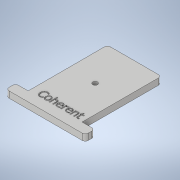
# Autodesk Inventor part: 00_Slider_Mask_DPC
Saved by Autodesk Inventor 2022 (Build 260153000, 153)
## iProperties
Created: 2021-10-22
Part Number: 00_Slider_Mask_DPC
Material: Generic
Document SubType Name: Modeling
Designer: diederichbenedict
Density: 1 g/cm^3
Appearance: Default
Author: diederichbenedict
Autodesk Inventor part; units mm, degrees
ref_plane "YZ Plane" through (0, 0, 0) normal (1, 0, 0) x (0, 1, 0)
ref_plane "XZ Plane" through (0, 0, 0) normal (0, 1, 0) x (-1, 0, 0)
ref_plane "XY Plane" through (0, 0, 0) normal (0, 0, 1) x (1, 0, 0)
sketch "Sketch1" plane through (0, 0, 0) normal (0, 1, 0) x (-1, 0, 0)
  line L0 (-17, 25) -> (17, 25)
  line L1 (17, 25) -> (17, -25)
  line L2 (17, -25) -> (-17, -25)
  line L3 (-17, -25) -> (-17, 25)
  line L4 (-17, 25) -> (17, -25) construction
  line L5 (17, 25) -> (-17, -25) construction
  line L6 (9, -17) -> (9, 17)
  line L7 (9, 17) -> (-9, 17)
  line L8 (-9, 17) -> (-9, -17)
  line L9 (-9, -17) -> (9, -17)
  line L10 (-25, 31) -> (25, 31)
  line L11 (25, 31) -> (25, 25)
  line L12 (25, 25) -> (-25, 25)
  line L13 (-25, 25) -> (-25, 31)
  line L14 (-25, 31) -> (25, 25) construction
  line L15 (25, 31) -> (-25, 25) construction
  point P0 (0, 0)
  point P1 (0, 28)
  point P2 (0, 25)
  dimension "d0" = 34
  dimension "d1" = 50
  dimension "d2" = 8
  dimension "d3" = 50
  dimension "d4" = 6
  constraints: 32 end point, 6 midpoint, 6 parallel, 3 perpendicular, 2 horizontal, 3 other
  measures "d0" distance of L1.end L2.end
  measures "d1" distance of L0.end L1.end
  measures "d2" distance between parallel lines of L1 L6
  measures "d3" distance of L11.end L12.end
  measures "d4" distance of L10.end L11.end
extrude "Extrusion1" add sketch "Sketch1" along normal blind 4 contours L12 L13 L10 L11 L0 | L0 L1 L2 L3 | L9 L8 L7 L6
sketch "Sketch2" plane through (0, 4, 0) normal (0, 1, 0) x (1, 0, 0)
  line L0 (25, -25) -> (17, -25) projected
  line L1 (17, -25) -> (17, 25) projected
  line L2 (17, 25) -> (-17, 25) projected
  line L3 (-17, 25) -> (-17, -25) projected
  line L4 (-17, -25) -> (-25, -25) projected
  line L5 (-25, -25) -> (-25, -31) projected
  line L6 (-25, -31) -> (25, -31) projected
  line L7 (25, -31) -> (25, -25) projected
  line L8 (13.5, 17) -> (-13.5, 17)
  line L9 (13.5, 17) -> (-13.5, -17) construction
  line L10 (-13.5, 17) -> (13.5, -17) construction
  circle A0 centre (0, 0.2783) radius 1.5
  point P0 (-1.4697, 0.3)
  point P1 (1.4697, 0.3)
  point P2 (-1.5, 0.2783)
  point P3 (1.5, 0.2783)
  dimension "d7" = 27
  dimension "d8" = 34
  dimension "d17" = 3
  constraints: 6 end point, 2 point on circle, 1 centre point, 1 horizontal
  measures "d7" distance of L10.end L9.end
  measures "d8" distance of L9.end L8.end
  measures "d17" diameter of A0
extrude "Extrusion2" cut sketch "Sketch2" against normal through all contours A0
sketch "Sketch3" plane through (0, 4, 0) normal (0, 1, 0) x (1, 0, 0)
  line L0 (-12.5562, -19.3436) -> (12.6697, -19.3436) construction
  line L1 (12.6697, -19.3436) -> (12.6697, -24.5308) construction
  line L2 (12.6697, -24.5308) -> (-12.5562, -24.5308) construction
  line L3 (-12.5562, -24.5308) -> (-12.5562, -19.3436) construction
  spline S0 degree 2 poles (-10.1618, -24.515) (-10.6351, -24.515) (-11.4359, -24.1955) (-11.7278, -23.876) knots 0 0 0 1 2 2 2
  spline S1 degree 2 poles (-11.7278, -23.876) (-12.0197, -23.5604) (-12.3392, -22.6137) (-12.3392, -21.9984) knots 0 0 0 1 2 2 2
  spline S2 degree 2 poles (-12.3392, -21.9984) (-12.3392, -21.387) (-12.0276, -20.4797) (-11.7317, -20.1444) knots 0 0 0 1 2 2 2
  spline S3 degree 2 poles (-11.7317, -20.1444) (-11.4398, -19.817) (-10.643, -19.4738) (-10.1499, -19.4738) knots 0 0 0 1 2 2 2
  spline S4 degree 2 poles (-10.1499, -19.4738) (-9.9054, -19.4738) (-9.4754, -19.5448) (-9.294, -19.6) knots 0 0 0 1 2 2 2
  spline S5 degree 2 poles (-9.294, -19.6) (-9.1362, -19.6513) (-8.8088, -19.7973) (-8.647, -19.8841) knots 0 0 0 1 2 2 2
  line L4 (-8.647, -19.8841) -> (-8.647, -20.6651)
  line L5 (-8.647, -20.6651) -> (-8.6983, -20.6651)
  spline S6 degree 2 poles (-8.6983, -20.6651) (-8.7851, -20.5862) (-9.0533, -20.3653) (-9.2466, -20.2588) knots 0 0 0 1 2 2 2
  spline S7 degree 2 poles (-9.2466, -20.2588) (-9.432, -20.1562) (-9.8699, -20.0261) (-10.1539, -20.0261) knots 0 0 0 1 2 2 2
  spline S8 degree 2 poles (-10.1539, -20.0261) (-10.4655, -20.0261) (-11.0217, -20.2825) (-11.2308, -20.527) knots 0 0 0 1 2 2 2
  spline S9 degree 2 poles (-11.2308, -20.527) (-11.4359, -20.7755) (-11.6647, -21.529) (-11.6647, -21.9984) knots 0 0 0 1 2 2 2
  spline S10 degree 2 poles (-11.6647, -21.9984) (-11.6647, -22.4993) (-11.4241, -23.2212) (-11.215, -23.4697) knots 0 0 0 1 2 2 2
  spline S11 degree 2 poles (-11.215, -23.4697) (-11.0099, -23.7103) (-10.4616, -23.9549) (-10.1539, -23.9549) knots 0 0 0 1 2 2 2
  spline S12 degree 2 poles (-10.1539, -23.9549) (-9.8738, -23.9549) (-9.3965, -23.8168) (-9.2111, -23.7143) knots 0 0 0 1 2 2 2
  spline S13 degree 2 poles (-9.2111, -23.7143) (-9.0336, -23.6117) (-8.7693, -23.3987) (-8.6944, -23.3238) knots 0 0 0 1 2 2 2
  line L6 (-8.6944, -23.3238) -> (-8.647, -23.3238)
  line L7 (-8.647, -23.3238) -> (-8.647, -24.0969)
  spline S14 degree 2 poles (-8.647, -24.0969) (-8.8088, -24.1719) (-9.0928, -24.3099) (-9.294, -24.373) knots 0 0 0 1 2 2 2
  spline S15 degree 2 poles (-9.294, -24.373) (-9.507, -24.444) (-9.8699, -24.515) (-10.1618, -24.515) knots 0 0 0 1 2 2 2
  spline S16 degree 2 poles (-5.089, -22.6019) (-5.089, -23.5249) (-5.9765, -24.5308) (-6.7181, -24.5308) knots 0 0 0 1 2 2 2
  spline S17 degree 2 poles (-6.7181, -24.5308) (-7.4794, -24.5308) (-8.3512, -23.4934) (-8.3512, -22.6019) knots 0 0 0 1 2 2 2
  spline S18 degree 2 poles (-8.3512, -22.6019) (-8.3512, -21.6868) (-7.4518, -20.673) (-6.7181, -20.673) knots 0 0 0 1 2 2 2
  spline S19 degree 2 poles (-6.7181, -20.673) (-5.9765, -20.673) (-5.089, -21.6828) (-5.089, -22.6019) knots 0 0 0 1 2 2 2
  spline S20 degree 2 poles (-5.7241, -22.6019) (-5.7241, -21.8919) (-6.2408, -21.2016) (-6.7181, -21.2016) knots 0 0 0 1 2 2 2
  spline S21 degree 2 poles (-6.7181, -21.2016) (-7.1954, -21.2016) (-7.7161, -21.8919) (-7.7161, -22.6019) knots 0 0 0 1 2 2 2
  spline S22 degree 2 poles (-7.7161, -22.6019) (-7.7161, -23.2922) (-7.1954, -24.0022) (-6.7181, -24.0022) knots 0 0 0 1 2 2 2
  spline S23 degree 2 poles (-6.7181, -24.0022) (-6.2448, -24.0022) (-5.7241, -23.304) (-5.7241, -22.6019) knots 0 0 0 1 2 2 2
  line L8 (-1.5901, -24.4283) -> (-2.2055, -24.4283)
  line L9 (-2.2055, -24.4283) -> (-2.2055, -22.3455)
  spline S24 degree 2 poles (-2.2055, -22.3455) (-2.2055, -22.093) (-2.2528, -21.6591) (-2.3238, -21.529) knots 0 0 0 1 2 2 2
  spline S25 degree 2 poles (-2.3238, -21.529) (-2.3988, -21.3909) (-2.667, -21.2568) (-2.8958, -21.2568) knots 0 0 0 1 2 2 2
  spline S26 degree 2 poles (-2.8958, -21.2568) (-3.1246, -21.2568) (-3.6098, -21.5014) (-3.8425, -21.6986) knots 0 0 0 1 2 2 2
  line L10 (-3.8425, -21.6986) -> (-3.8425, -24.4283)
  line L11 (-3.8425, -24.4283) -> (-4.4579, -24.4283)
  line L12 (-4.4579, -24.4283) -> (-4.4579, -19.3436)
  line L13 (-4.4579, -19.3436) -> (-3.8425, -19.3436)
  line L14 (-3.8425, -19.3436) -> (-3.8425, -21.1818)
  spline S27 degree 2 poles (-3.8425, -21.1818) (-3.5664, -20.9333) (-3.0339, -20.673) (-2.7341, -20.673) knots 0 0 0 1 2 2 2
  spline S28 degree 2 poles (-2.7341, -20.673) (-2.1976, -20.673) (-1.5901, -21.383) (-1.5901, -22.0575) knots 0 0 0 1 2 2 2
  line L15 (-1.5901, -22.0575) -> (-1.5901, -24.4283)
  spline S29 degree 2 poles (0.8595, -24.5111) (-0.0162, -24.5111) (-0.9787, -23.5289) (-0.9787, -22.6216) knots 0 0 0 1 2 2 2
  spline S30 degree 2 poles (-0.9787, -22.6216) (-0.9787, -21.7301) (-0.0438, -20.673) (0.7096, -20.673) knots 0 0 0 1 2 2 2
  spline S31 degree 2 poles (0.7096, -20.673) (1.0488, -20.673) (1.5735, -20.8702) (1.7667, -21.0793) knots 0 0 0 1 2 2 2
  spline S32 degree 2 poles (1.7667, -21.0793) (1.964, -21.2883) (2.173, -21.8919) (2.173, -22.3297) knots 0 0 0 1 2 2 2
  line L16 (2.173, -22.3297) -> (2.173, -22.665)
  line L17 (2.173, -22.665) -> (-0.3555, -22.665)
  spline S33 degree 2 poles (-0.3555, -22.665) (-0.3555, -23.3001) (0.2836, -23.9746) (0.8516, -23.9746) knots 0 0 0 1 2 2 2
  spline S34 degree 2 poles (0.8516, -23.9746) (1.0528, -23.9746) (1.4433, -23.8839) (1.6011, -23.8129) knots 0 0 0 1 2 2 2
  spline S35 degree 2 poles (1.6011, -23.8129) (1.7667, -23.734) (1.9955, -23.5959) (2.0705, -23.5328) knots 0 0 0 1 2 2 2
  line L18 (2.0705, -23.5328) -> (2.106, -23.5328)
  line L19 (2.106, -23.5328) -> (2.106, -24.2034)
  spline S36 degree 2 poles (2.106, -24.2034) (1.9995, -24.2468) (1.676, -24.373) (1.5498, -24.4085) knots 0 0 0 1 2 2 2
  spline S37 degree 2 poles (1.5498, -24.4085) (1.3723, -24.4598) (1.0804, -24.5111) (0.8595, -24.5111) knots 0 0 0 1 2 2 2
  spline S38 degree 2 poles (1.5735, -22.1956) (1.5656, -21.9471) (1.463, -21.5842) (1.3644, -21.4619) knots 0 0 0 1 2 2 2
  spline S39 degree 2 poles (1.3644, -21.4619) (1.2579, -21.3238) (0.9226, -21.1779) (0.6741, -21.1779) knots 0 0 0 1 2 2 2
  spline S40 degree 2 poles (0.6741, -21.1779) (0.4295, -21.1779) (0.0863, -21.3238) (-0.0557, -21.4659) knots 0 0 0 1 2 2 2
  spline S41 degree 2 poles (-0.0557, -21.4659) (-0.1937, -21.6118) (-0.3357, -21.9629) (-0.3555, -22.1956) knots 0 0 0 1 2 2 2
  line L20 (-0.3555, -22.1956) -> (1.5735, -22.1956)
  line L21 (4.7331, -21.4343) -> (4.7015, -21.4343)
  spline S42 degree 2 poles (4.7015, -21.4343) (4.6305, -21.4146) (4.4767, -21.4067) (4.3702, -21.4067) knots 0 0 0 1 2 2 2
  spline S43 degree 2 poles (4.3702, -21.4067) (4.1217, -21.4067) (3.6325, -21.6236) (3.4116, -21.8366) knots 0 0 0 1 2 2 2
  line L22 (3.4116, -21.8366) -> (3.4116, -24.4283)
  line L23 (3.4116, -24.4283) -> (2.7963, -24.4283)
  line L24 (2.7963, -24.4283) -> (2.7963, -20.7755)
  line L25 (2.7963, -20.7755) -> (3.4116, -20.7755)
  line L26 (3.4116, -20.7755) -> (3.4116, -21.3199)
  spline S44 degree 2 poles (3.4116, -21.3199) (3.7469, -21.0201) (4.2479, -20.7755) (4.4846, -20.7755) knots 0 0 0 1 2 2 2
  spline S45 degree 2 poles (4.4846, -20.7755) (4.5792, -20.7755) (4.6739, -20.7834) (4.7331, -20.7953) knots 0 0 0 1 2 2 2
  line L27 (4.7331, -20.7953) -> (4.7331, -21.4343)
  spline S46 degree 2 poles (6.7961, -24.5111) (5.9204, -24.5111) (4.9579, -23.5289) (4.9579, -22.6216) knots 0 0 0 1 2 2 2
  spline S47 degree 2 poles (4.9579, -22.6216) (4.9579, -21.7301) (5.8928, -20.673) (6.6462, -20.673) knots 0 0 0 1 2 2 2
  spline S48 degree 2 poles (6.6462, -20.673) (6.9855, -20.673) (7.5101, -20.8702) (7.7034, -21.0793) knots 0 0 0 1 2 2 2
  spline S49 degree 2 poles (7.7034, -21.0793) (7.9006, -21.2883) (8.1097, -21.8919) (8.1097, -22.3297) knots 0 0 0 1 2 2 2
  line L28 (8.1097, -22.3297) -> (8.1097, -22.665)
  line L29 (8.1097, -22.665) -> (5.5812, -22.665)
  spline S50 degree 2 poles (5.5812, -22.665) (5.5812, -23.3001) (6.2202, -23.9746) (6.7882, -23.9746) knots 0 0 0 1 2 2 2
  spline S51 degree 2 poles (6.7882, -23.9746) (6.9894, -23.9746) (7.3799, -23.8839) (7.5377, -23.8129) knots 0 0 0 1 2 2 2
  spline S52 degree 2 poles (7.5377, -23.8129) (7.7034, -23.734) (7.9322, -23.5959) (8.0071, -23.5328) knots 0 0 0 1 2 2 2
  line L30 (8.0071, -23.5328) -> (8.0426, -23.5328)
  line L31 (8.0426, -23.5328) -> (8.0426, -24.2034)
  spline S53 degree 2 poles (8.0426, -24.2034) (7.9361, -24.2468) (7.6127, -24.373) (7.4864, -24.4085) knots 0 0 0 1 2 2 2
  spline S54 degree 2 poles (7.4864, -24.4085) (7.3089, -24.4598) (7.017, -24.5111) (6.7961, -24.5111) knots 0 0 0 1 2 2 2
  spline S55 degree 2 poles (7.5101, -22.1956) (7.5022, -21.9471) (7.3996, -21.5842) (7.301, -21.4619) knots 0 0 0 1 2 2 2
  spline S56 degree 2 poles (7.301, -21.4619) (7.1945, -21.3238) (6.8592, -21.1779) (6.6107, -21.1779) knots 0 0 0 1 2 2 2
  spline S57 degree 2 poles (6.6107, -21.1779) (6.3662, -21.1779) (6.023, -21.3238) (5.881, -21.4659) knots 0 0 0 1 2 2 2
  spline S58 degree 2 poles (5.881, -21.4659) (5.7429, -21.6118) (5.6009, -21.9629) (5.5812, -22.1956) knots 0 0 0 1 2 2 2
  line L32 (5.5812, -22.1956) -> (7.5101, -22.1956)
  line L33 (11.6007, -24.4283) -> (10.9853, -24.4283)
  line L34 (10.9853, -24.4283) -> (10.9853, -22.3455)
  spline S59 degree 2 poles (10.9853, -22.3455) (10.9853, -22.093) (10.938, -21.6591) (10.867, -21.529) knots 0 0 0 1 2 2 2
  spline S60 degree 2 poles (10.867, -21.529) (10.792, -21.3909) (10.5238, -21.2568) (10.295, -21.2568) knots 0 0 0 1 2 2 2
  spline S61 degree 2 poles (10.295, -21.2568) (10.0662, -21.2568) (9.581, -21.5014) (9.3483, -21.6986) knots 0 0 0 1 2 2 2
  line L35 (9.3483, -21.6986) -> (9.3483, -24.4283)
  line L36 (9.3483, -24.4283) -> (8.7329, -24.4283)
  line L37 (8.7329, -24.4283) -> (8.7329, -20.7755)
  line L38 (8.7329, -20.7755) -> (9.3483, -20.7755)
  line L39 (9.3483, -20.7755) -> (9.3483, -21.1818)
  spline S62 degree 2 poles (9.3483, -21.1818) (9.6244, -20.9333) (10.1569, -20.673) (10.4567, -20.673) knots 0 0 0 1 2 2 2
  spline S63 degree 2 poles (10.4567, -20.673) (10.9932, -20.673) (11.6007, -21.383) (11.6007, -22.0575) knots 0 0 0 1 2 2 2
  line L40 (11.6007, -22.0575) -> (11.6007, -24.4283)
  spline S64 degree 2 poles (13.569, -24.4993) (13.0681, -24.4993) (12.504, -23.9273) (12.504, -23.308) knots 0 0 0 1 2 2 2
  line L41 (12.504, -23.308) -> (12.504, -21.2844)
  line L42 (12.504, -21.2844) -> (12.0898, -21.2844)
  line L43 (12.0898, -21.2844) -> (12.0898, -20.7755)
  line L44 (12.0898, -20.7755) -> (12.504, -20.7755)
  line L45 (12.504, -20.7755) -> (12.504, -19.7263)
  line L46 (12.504, -19.7263) -> (13.1193, -19.7263)
  line L47 (13.1193, -19.7263) -> (13.1193, -20.7755)
  line L48 (13.1193, -20.7755) -> (14.2514, -20.7755)
  line L49 (14.2514, -20.7755) -> (14.2514, -21.2844)
  line L50 (14.2514, -21.2844) -> (13.1193, -21.2844)
  line L51 (13.1193, -21.2844) -> (13.1193, -23.024)
  spline S65 degree 2 poles (13.1193, -23.024) (13.1193, -23.3001) (13.1391, -23.6038) (13.2061, -23.734) knots 0 0 0 1 2 2 2
  spline S66 degree 2 poles (13.2061, -23.734) (13.2613, -23.8484) (13.5099, -23.9628) (13.7229, -23.9628) knots 0 0 0 1 2 2 2
  spline S67 degree 2 poles (13.7229, -23.9628) (13.8728, -23.9628) (14.1528, -23.8721) (14.2159, -23.8445) knots 0 0 0 1 2 2 2
  line L52 (14.2159, -23.8445) -> (14.2514, -23.8445)
  line L53 (14.2514, -23.8445) -> (14.2514, -24.3967)
  spline S68 degree 2 poles (14.2514, -24.3967) (14.0779, -24.444) (13.7229, -24.4993) (13.569, -24.4993) knots 0 0 0 1 2 2 2
  point P0 (0, 0)
  constraints: 2 other
extrude "Extrusion3" cut sketch "Sketch3" against normal blind 1
fillet "Fillet1" radius 2 6 edges at (25, 2, 31) (25, 2, 25) (-25, 2, 31) (-25, 2, 25) (-17, 2, -25) (17, 2, -25)
body "Solid1"
